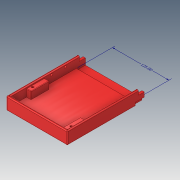
# Autodesk Inventor part: Case_metà1
Saved by Autodesk Inventor 2019 (Build 230136000, 136)
## iProperties
Created: 2019-05-06
Part Number: Case_metà1
Material: Generic
Document SubType Name: Modeling
Designer: giacomo
Density: 1 g/cm^3
Appearance: Light Red
Author: giacomo
Autodesk Inventor part; units mm, degrees
ref_plane "YZ Plane" through (0, 0, 0) normal (1, 0, 0) x (0, 1, 0)
ref_plane "XZ Plane" through (0, 0, 0) normal (0, 1, 0) x (-1, 0, 0)
sketch "Sketch1" plane through (0, 0, 0) normal (0, 1, 0) x (-1, 0, 0)
  line L0 (-67.5, 75) -> (67.5, 75)
  line L1 (67.5, 75) -> (67.5, -75)
  line L2 (67.5, -75) -> (-67.5, -75)
  line L3 (-67.5, -75) -> (-67.5, 75)
  line L4 (-67.5, 75) -> (67.5, -75) construction
  line L5 (67.5, 75) -> (-67.5, -75) construction
  point P0 (0, 0)
  dimension "d0" = 135
  dimension "d1" = 150
  constraints: 12 end point, 2 midpoint, 2 parallel, 1 horizontal, 1 perpendicular
  measures "d0" distance of L1.end L2.end
  measures "d1" distance of L0.end L1.end
extrude "Extrusion1" add sketch "Sketch1" along normal blind 8
sketch "Sketch3" plane through (0, 8, 0) normal (0, 1, 0) x (1, 0, 0)
  line L0 (-67.5, -75) -> (67.5, -75) projected
  line L1 (67.5, -75) -> (67.5, 75) projected
  line L2 (67.5, 75) -> (-67.5, 75) projected
  line L3 (-67.5, 75) -> (-67.5, -75) projected
  line L4 (62.5, 75) -> (62.5, -70)
  line L5 (-67.5, -75) -> (67.5, -75) projected
  line L6 (67.5, -75) -> (67.5, 75) projected
  line L7 (0, 0) -> (0, -83) construction
  line L8 (-62.5, 75) -> (-62.5, -70)
  line L9 (62.5, -70) -> (-62.5, -70)
  dimension "d4" = 5
  dimension "d5" = 5
  constraints: 8 end point, 3 parallel, 2 point on line, 1 perpendicular, 1 vertical, 1 other
  measures "d4" distance between parallel lines of L1 L4
  measures "d5" distance between parallel lines of L9 L0
extrude "Extrusion2" add sketch "Sketch3" along normal blind 20 contours L3 L2 L8 L9 L4 L1 L0
sketch "Sketch4" plane through (67.5, 0, -75) normal (0, 0, -1) x (-1, 0, 0)
  line L0 (135, 0) -> (0, 0) projected
  line L1 (135, 0) -> (135, 28) projected
  line L2 (130, 28) -> (135, 28) projected
  line L3 (130, 8) -> (130, 28) projected
  line L4 (5, 8) -> (130, 8) projected
  line L5 (5, 8) -> (5, 28) projected
  line L6 (0, 28) -> (5, 28) projected
  line L7 (0, 0) -> (0, 28) projected
  line L8 (130, 8) -> (5, 8) projected
  line L9 (5, 8) -> (5, 0)
  line L10 (130, 8) -> (130, 0)
  line L11 (0, 0) -> (135, 0) projected
  line L12 (0, 0) -> (0, 28) projected
  line L13 (5, 0) -> (130, 0)
  line L14 (5, 8) -> (130, 8) projected
  line L15 (5, 4) -> (130, 4)
  line L16 (5, 8) -> (0, 8)
  line L17 (135, 0) -> (0, 0) projected
  point P0 (67.5, 0)
  dimension "d8" = 0
  dimension "d9" = 4
  constraints: 10 end point, 6 parallel, 6 point on line, 2 midpoint, 2 perpendicular, 1 vertical
  measures "d8" distance between parallel lines of L0 L13
  measures "d9" distance between parallel lines of L13 L15
extrude "Extrusion3" add sketch "Sketch4" along normal blind 20 contours L0 L10 L3 L2 L1 | L0 L9 L15 L10 | L15 L9 L4 L10 | L7 L6 L5 L16
sketch "Sketch6" plane through (67.5, 0, 75) normal (1, 0, 0) x (0, 0, -1)
  line L0 (150, 0) -> (150, 8)
  line L1 (0, 0) -> (0, 28) projected
  line L2 (170, 18) -> (157, 18)
  line L3 (157, 18) -> (157, 28)
  line L4 (157, 28) -> (170, 28)
  line L5 (170, 28) -> (170, 18)
  line L6 (170, 28) -> (170, 8) projected
  line L7 (150, 8) -> (170, 8) projected
  line L8 (0, 28) -> (170, 28) projected
  point P0 (75, 0)
  dimension "d83" = 10
  dimension "d85" = 10
  dimension "d86" = 0
  dimension "d87" = 13
  dimension "d88" = 0
  dimension "d89" = 0
  constraints: 10 end point, 1 collinear, 1 vertical
  measures "d83" distance from line of L7 L2.start
  measures "d85" distance of L4.end L2.start
  measures "d86" distance between parallel lines of L6 L5
  measures "d87" distance between parallel lines of L5 L3
  measures "d88" vertical distance of L3.end L4.end
  measures "d89" vertical distance of L2.end L2.start
extrude "Extrusion4" cut sketch "Sketch6" against normal through all
fillet "Fillet1" radius 2 11 edges at (67.5, 0, 0) (67.5, 28, -3.5) (67.5, 14, 75) (0, 28, 75) (0, 0, 75) (-67.5, 28, -3.5) (-67.5, 14, 75) (-67.5, 0, -10) (62.5, 28, -6) (-62.5, 28, -6) (0, 28, 70)
sketch "Sketch11" plane through (-67.5, 9.7, -88) normal (-1, 0, 0) x (0, 0, 1)
  line L0 (9, 17.5) -> (0, 19.5) projected
  line L1 (0, 19.5) -> (0, 11.5) projected
  line L2 (0, 11.5) -> (9, 14) projected
  line L3 (9, 17.5) -> (9, 14) projected
  line L4 (9, 6) -> (0, 8.5) projected
  line L5 (0, 0) -> (9, 2.5) projected
  line L6 (0, 6) -> (0, 0) projected
  line L7 (9, 6) -> (9, 2.5) projected
  point P0 (88, -9.7)
sketch "Sketch12" plane through (-67.5, 2, 73) normal (-1, 0, 0) x (0, 0, 1)
  line L0 (-168, 28) -> (-168, 20)
  line L1 (-159, 26) -> (-168, 28)
  line L2 (-159, 26) -> (-159, 22.5)
  line L3 (-168, 20) -> (-159, 22.5)
  line L4 (-168, 17) -> (-168, 8.5)
  line L5 (-159, 14.5) -> (-168, 17)
  line L6 (-159, 14.5) -> (-159, 11)
  line L7 (-168, 8.5) -> (-159, 11)
  line L8 (-168, 0) -> (-168, 16) projected
  line L9 (-161, 19.2) -> (-161, 27.2) projected
  line L10 (-161, 27.2) -> (-168, 27.2)
  line L11 (-168, 16) -> (-168, 6) projected
  line L12 (-159, 17) -> (-168, 17)
  point P0 (-73, -2)
  point P1 (-168, 24)
  constraints: 20 end point, 2 perpendicular, 2 point on line
sketch "Sketch15" plane through (62.5, 6, -75) normal (1, 0, 0) x (0, 0, -1)
  line L0 (0, -6) -> (0, 2) projected
  line L1 (20, 2) -> (20, -6) projected
  line L2 (0, 2) -> (20, 2) projected
  line L3 (0, -6) -> (20, -6) projected
  point P0 (-75, -6)
extrude "Extrusion8" add sketch "Sketch15" along normal blind 2.5
sketch "Sketch16" plane through (0, 8, 0) normal (0, 1, 0) x (1, 0, 0)
  line L0 (-62.5, -35) -> (-52.5, -35)
  line L1 (-52.5, -35) -> (-52.5, 5)
  line L2 (-52.5, 5) -> (-62.5, 5)
  line L3 (-62.5, 5) -> (-62.5, -35)
  line L4 (62.5, -70) -> (-62.5, -70) projected
  line L5 (-62.5, -70) -> (-62.5, 82) projected
  line L6 (51.5, -70) -> (62.5, -70)
  line L7 (62.5, -70) -> (62.5, -30)
  line L8 (62.5, -30) -> (51.5, -30)
  line L9 (51.5, -30) -> (51.5, -70)
  line L10 (62.5, 82) -> (62.5, -70) projected
  point P0 (0, 0)
  point P1 (-62.5, 95)
  point P2 (62.5, 95)
  dimension "d39" = 35
  dimension "d40" = 0
  dimension "d41" = 10
  dimension "d42" = 40
  dimension "d43" = 0
  dimension "d44" = 0
  dimension "d45" = 40
  dimension "d46" = 11
  constraints: 16 end point, 4 parallel, 2 horizontal, 2 perpendicular
  measures "d39" distance between parallel lines of L4 L0
  measures "d40" distance between parallel lines of L5 L3
  measures "d41" distance between parallel lines of L1 L3
  measures "d42" distance of L0.end L1.end
  measures "d43" distance between parallel lines of L4 L6
  measures "d44" distance between parallel lines of L10 L7
  measures "d45" distance of L8.end L6.start
  measures "d46" distance of L7.end L8.end
extrude "Extrusion9" add sketch "Sketch16" along normal blind 16
fillet "Fillet4" radius 1 8 edges at (51.5, 24, 50) (57, 24, 30) (51.5, 16, 30) (-52.5, 24, 15) (-52.5, 16, -5) (-57.5, 24, 35) (-57.5, 24, -5) (-52.5, 16, 35)
sketch "Sketch17" plane through (0, 24, 0) normal (0, 1, 0) x (1, 0, 0)
  circle A0 centre (-59, -25) radius 2.25
  line L0 (-62.5, -34) -> (-62.5, 4) projected
  line L1 (-53.5, -34) -> (-62.5, -34) projected
  circle A1 centre (58.5, -57.5) radius 2.25
  line L2 (52.5, -70) -> (52.5, -31) projected
  line L3 (52.5, -31) -> (62.5, -31) projected
  line L4 (62.5, -70) -> (50.5, -70) projected
  point P0 (0, 0)
  dimension "d50" = 4.5
  dimension "d51" = 3.5
  dimension "d52" = 9
  dimension "d53" = 4.5
  dimension "d54" = 6
  dimension "d90" = 12.5
  constraints: 2 centre point, 1 other
  measures "d50" diameter of A0
  measures "d51" distance from line of L0 A0.centre
  measures "d52" distance from line of L1 A0.centre
  measures "d53" diameter of A1
  measures "d90" distance from line of L4 A1.centre
extrude "Extrusion10" cut sketch "Sketch17" against normal blind 12
sketch "Sketch18" plane through (-62.5, 9.7, -88) normal (1, 0, 0) x (0, 0, -1)
  circle A0 centre (-68, 13.3) radius 2.25
  circle A1 centre (-37.2, 13.3) radius 2.25
  line L0 (0, 8.1) -> (0, 14.1)
  line L1 (-37.2, 13.3) -> (-68, 13.3)
  line L2 (-6, 18.3) -> (-160, 18.3) projected
  line L3 (-158, -1.7) -> (-158, 16.3) projected
  point P0 (-88, -9.7)
  point P1 (7, 18.3)
  dimension "d60" = 4.5
  dimension "d61" = 4.5
  dimension "d62" = 30.8
  dimension "d64" = 5
  dimension "d67" = 90
  constraints: 4 end point, 2 centre point, 1 horizontal
  measures "d60" diameter of A0
  measures "d61" diameter of A1
  measures "d62" distance of L1.start L1.end
  measures "d64" distance between parallel lines of L1 L2
  measures "d67" distance from line of L3 L1.end
extrude "Extrusion11" cut sketch "Sketch18" against normal through all
ref_plane "Work Plane3" through (0, 22.5, 0) normal (0, 1, 0) x (1, 0, 0)
sketch "Sketch21" plane through (0, 22.5, 0) normal (0, 1, 0) x (1, 0, 0)
  circle A0 centre (58.5, -57.5) radius 2.25 projected
  line L0 (54.75, -55.3349) -> (58.5, -53.1699)
  line L1 (58.5, -53.1699) -> (62.25, -55.3349)
  line L2 (62.25, -55.3349) -> (62.25, -59.6651)
  line L3 (62.25, -59.6651) -> (58.5, -61.8301)
  line L4 (58.5, -61.8301) -> (54.75, -59.6651)
  line L5 (54.75, -59.6651) -> (54.75, -55.3349)
  line L6 (-62.5, -35) -> (-62.5, -70) projected
  line L7 (51.5, -70) -> (51.5, -31) projected
  circle A1 centre (-59, -25) radius 2.25 projected
  line L8 (-55.25, -27.1651) -> (-59, -29.3301)
  line L9 (-59, -29.3301) -> (-62.75, -27.1651)
  line L10 (-62.75, -27.1651) -> (-62.75, -22.8349)
  line L11 (-62.75, -22.8349) -> (-59, -20.6699)
  line L12 (-59, -20.6699) -> (-55.25, -22.8349)
  line L13 (-55.25, -22.8349) -> (-55.25, -27.1651)
  point P0 (0, 0)
  dimension "d78" = 7.5
  dimension "d79" = 7.5
  constraints: 24 end point, 2 coincident, 2 parallel, 26 other
  measures "d78" distance between parallel lines of L2 L5
  measures "d79" distance between parallel lines of L13 L10
extrude "Extrusion13" cut sketch "Sketch21" against normal blind 3.15
sketch "Sketch22" plane through (0, 8, 0) normal (0, 1, 0) x (1, 0, 0)
  line L0 (65, 75) -> (65, 95) projected
  line L1 (-62.5, 95) -> (62.5, 95) projected
  line L2 (65, 75) -> (67.5, 75) projected
  line L3 (-62.5, 95) -> (65, 95)
  line L4 (65, 95) -> (65, 75)
  line L5 (65, 75) -> (-62.5, 75)
  line L6 (-62.5, 75) -> (-62.5, 95)
  point P0 (0, 0)
  constraints: 8 end point, 2 parallel, 1 horizontal, 1 perpendicular
extrude "Extrusion14" cut sketch "Sketch22" against normal blind 4
sketch "Sketch23" plane through (65, 6, -75) normal (1, 0, 0) x (0, 0, -1)
  line L0 (20, -2) -> (0, -2) projected
  line L1 (0, -6) -> (0, -2) projected
  line L2 (0, -6) -> (20, -6) projected
  line L3 (20, -6) -> (20, -2) projected
  point P0 (-75, -6)
extrude "Extrusion15" cut sketch "Sketch23" against normal up to surface (2.5 mm away)
body "Solid1"
